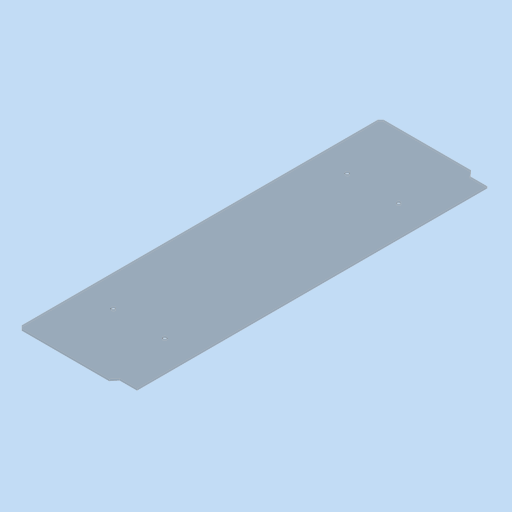
# Autodesk Inventor part: enc-BackPanel Top for 4040
Saved by Autodesk Inventor 2023.2 (Build 272271000, 271)
## iProperties
Created: 2023-12-04
Part Number: enc-BackPanel Top for 4040
Material: Generisch
Document SubType Name: Modeling
Designer: Nils Bade
Density: 1 g/cm^3
Appearance: PVC Verglasung
Author: Nils Bade
Autodesk Inventor part; units mm, degrees
ref_plane "YZ Plane" through (0, 0, 0) normal (1, 0, 0) x (0, 1, 0)
ref_plane "XZ Plane" through (0, 0, 0) normal (0, 1, 0) x (-1, 0, 0)
ref_plane "XY Plane" through (0, 0, 0) normal (0, 0, 1) x (1, 0, 0)
sketch "Skizze1" plane through (0, 0, 0) normal (0, 1, 0) x (-1, 0, 0)
  line L0 (97.5, 314) -> (-97.5, 314)
  line L1 (-97.5, 314) -> (-97.5, -314)
  line L2 (-97.5, -314) -> (97.5, -314)
  line L3 (97.5, -314) -> (97.5, 314)
  line L4 (97.5, 314) -> (-97.5, -314) construction
  line L5 (-97.5, 314) -> (97.5, -314) construction
  line L6 (-136.5, 0) -> (136.5, 0) construction
  line L7 (0, -439.6) -> (0, 439.6) construction
  circle A0 centre (44.5, -203) radius 3.25
  circle A1 centre (-44.5, -203) radius 3.25
  circle A2 centre (44.5, 203) radius 3.25
  circle A3 centre (-44.5, 203) radius 3.25
  line L8 (-59, -314) -> (-67.391, -304)
  line L9 (-67.391, -304) -> (-97.5, -304)
  line L10 (-59, 314) -> (-67.391, 304)
  line L11 (-67.391, 304) -> (-97.5, 304)
  point P0 (0, 0)
  dimension "d0" = 628
  dimension "d1" = 195
  dimension "d2" = 6.5
  dimension "d3" = 44.5
  dimension "d4" = 111
  dimension "d10" = 38.5
  dimension "d11" = 10
  dimension "d12" = 50
  constraints: 20 end point, 6 symmetric about line, 4 centre point, 2 midpoint, 2 parallel, 2 perpendicular, 2 point on line, 1 horizontal, 3 other
  measures "d0" distance of L2.end L0.start
  measures "d1" distance of L1.end L2.end
  measures "d2" diameter of A0
  measures "d3" distance from line of L7 A0.centre
  measures "d4" distance from line of L2 A0.centre
  measures "d10" distance from line of L1 L8.start
  measures "d11" distance between parallel lines of L2 L9
  measures "d12" angle of L2 L8
extrude "Extrusion1" add sketch "Skizze1" along normal blind 3 contours L3 L2 L8 L9 L1 L11 L10 L0
chamfer "Fase1" distance 5 angle 45 2 edges at (-97.5, 1.5, 314) (-97.5, 1.5, -314)
